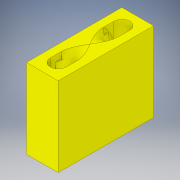
# Autodesk Inventor part: gripper
Saved by Autodesk Inventor 2019 (Build 230136000, 136)
## iProperties
Created: 2019-02-02
Part Number: gripper
Material: Generic
Document SubType Name: Modeling
Designer: suchanek
Density: 1 g/cm^3
Appearance: Default
Author: suchanek
Autodesk Inventor part; units mm, degrees
ref_plane "YZ Plane" through (0, 0, 0) normal (1, 0, 0) x (0, 1, 0)
ref_plane "XZ Plane" through (0, 0, 0) normal (0, 1, 0) x (-1, 0, 0)
ref_plane "XY Plane" through (0, 0, 0) normal (0, 0, 1) x (1, 0, 0)
sketch "Sketch1" plane through (0, 0, 0) normal (0, 1, 0) x (-1, 0, 0)
  line L0 (-5, 15) -> (5, 15)
  line L1 (5, 15) -> (5, -15)
  line L2 (5, -15) -> (-5, -15)
  line L3 (-5, -15) -> (-5, 15)
  line L4 (-5, 15) -> (5, -15) construction
  line L5 (5, 15) -> (-5, -15) construction
  circle A0 centre (0, 10) radius 2.5
  circle A1 centre (0, -10) radius 2.5
  line L6 (0, 0) -> (-2.5, 0)
  dimension "d0" = 10
  dimension "d1" = 30
  dimension "d2" = 5
  dimension "d4" = 20
  constraints: 14 end point, 3 midpoint, 2 centre point, 2 horizontal, 2 parallel, 1 perpendicular, 1 vertical alignment, 1 other
  measures "d0" distance of L1.end L2.end
  measures "d1" distance of L0.end L1.end
  measures "d2" diameter of A0
  measures "d4" distance of A1.centre A0.centre
extrude "Extrusion1" add sketch "Sketch1" along normal blind 25
sketch "Sketch2" plane through (0, 0, 0) normal (1, 0, 0) x (0, 1, 0)
  line L0 (0, 7.5) -> (0, 12.5)
  line L1 (0, 10) -> (17.5, 10)
  arc A0 (19.608122, -9.775266) -> (17.5, 10) centre (17.5, 0) ccw
  line L2 (19.608122, -9.775266) -> (0, -9.775266)
  line L3 (0, -12.5) -> (0, -7.5)
  line L4 (25, 12.5) -> (25, 7.5)
  point P0 (0, 0)
  dimension "d7" = 10
  dimension "d8" = 7.5
  constraints: 4 end point, 2 horizontal, 2 point on circle, 1 centre point, 1 midpoint, 1 point on line, 1 tangent
  measures "d7" radius of A0
  measures "d8" distance from line of L4 A0.centre
sketch "Sketch3" plane through (0, 0, 0) normal (0, -1, 0) x (1, 0, 0)
  circle A0 centre (0, 10) radius 2.5
  circle A1 centre (0, 10) radius 2.5 projected
  point P0 (0, 0)
  constraints: 2 concentric, 1 centre point
sweep "Sweep1" cut profiles "Sketch3" path "Sketch2" path curves L1 A0 L2
sketch "Sketch4" plane through (0, 25, 0) normal (0, 1, 0) x (1, 0, 0)
  arc A0 (-2.066993, -8.59375) -> (2.066993, -8.59375) centre (0, -10) ccw
  line L0 (2.5, -6.614378) -> (2.5, -10)
  line L1 (-2.5, -10) -> (2.5, -10)
  line L2 (2.5, -10) -> (2.5, -6.614378)
  line L3 (2.5, -6.614378) -> (-2.5, -6.614378)
  line L4 (-2.5, -6.614378) -> (-2.5, -10)
  line L5 (2.5, 9.775266) -> (2.5, 6.614378)
  arc A1 (-2.497473, 9.887633) -> (2.497473, 9.887633) centre (0, 9.775266) ccw
  line L6 (2.5, 6.614378) -> (-2.497473, 6.614378)
  line L7 (-2.497473, 6.614378) -> (-2.497473, 9.887633)
  line L8 (-2.497473, 9.887633) -> (2.5, 9.887633)
  line L9 (2.5, 9.887633) -> (2.5, 6.614378)
  spline S0 degree 5 poles (-2.066993, -8.59375) (-2.403323, -7.937602) (-2.559371, -7.182512) (-2.56244, -6.424204) (-2.463104, -5.675997) (-2.124369, -4.293412) (-1.902463, -3.656535) (-1.636985, -3.036469) (-1.342312, -2.43142) (-0.832449, -1.463374) (-0.629126, -1.094924) (-0.420997, -0.729057) (-0.210551, -0.364626) (-0.000277, -0.000482) (-0.000238, -0.000415) (-0.000199, -0.000347) (-0.00016, -0.000279) (-0.000121, -0.000212) (-0.00008, -0.000145) (-0.00007, -0.00011) (-0.000048, -0.000079) (-0.000024, -0.000055) (-0.000005, -0.000041) (0.000001, -0.000041) knots 0 0 0 0 0 0 0.26707586 0.26707586 0.26707586 0.26707586 0.50503941 0.50503941 0.50503941 0.50503941 0.65367347 0.65367347 0.65367347 0.65367347 0.65367347 0.82541871 0.82541871 0.82541871 0.82541871 0.82541871 1 1 1 1 1 1
  constraints: 16 end point, 4 parallel, 2 horizontal, 2 perpendicular, 2 point on line, 1 point on circle, 1 tangent, 4 other
sketch "Sketch4 outline for Extrusion2" plane through (0, 25, 0) normal (0, 1, 0) x (1, 0, 0)
  line L0 (-2.497473, 6.614378) -> (2.5, 6.614378)
  line L1 (-2.497473, 9.887633) -> (-2.497473, 6.614378)
  line L2 (2.5, 9.887633) -> (-2.497473, 9.887633)
  line L3 (2.5, 6.614378) -> (2.5, 9.887633)
  line L4 (2.5, -10) -> (2.5, -6.614378)
  line L5 (2.5, -6.614378) -> (-2.5, -6.614378)
  line L6 (-2.5, -6.614378) -> (-2.5, -10)
  line L7 (-2.5, -10) -> (2.5, -10)
extrude "Extrusion2" cut sketch "Sketch4 outline for Extrusion2" against normal blind 2
sketch "Sketch5" plane through (0, 23, 0) normal (0, 1, 0) x (1, 0, 0)
  arc A0 (2.5, -10) -> (-2.5, -10) centre (0, -10) ccw
  line L0 (2.5, -10) -> (-2.5, -10)
  line L1 (-2.5, -10) -> (-2.5, -8.351647)
  line L2 (-2.5, -8.351647) -> (2.5, -8.351647)
  line L3 (2.5, -8.351647) -> (2.5, -10)
  arc A1 (-2.497473, 9.887633) -> (2.497473, 9.887633) centre (0, 9.775266) ccw
  line L4 (-2.497473, 9.887633) -> (2.5, 9.887633)
  line L5 (2.5, 9.887633) -> (2.5, 8.351647)
  line L6 (2.5, 8.351647) -> (-2.497473, 8.351647)
  line L7 (-2.497473, 8.351647) -> (-2.497473, 9.887633)
  arc A2 (2.497473, 9.887633) -> (-2.497473, 9.887633) centre (0, 10) ccw
  point P0 (0, 0)
  constraints: 16 end point, 4 parallel, 2 horizontal, 2 perpendicular, 1 tangent, 4 other
extrude "Extrusion3" cut sketch "Sketch5" against normal blind 3 contours L0 A0 L2 | A0 L2 L3 | L1 L2 A0 | L4 A1 L6 | A1 L6 L7 | L4 L5 A1 | A1 L5 L6
body "Solid1"
